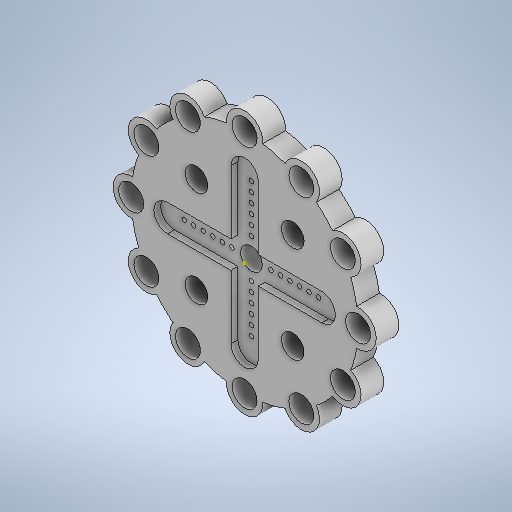
# Autodesk Inventor part: Servo_przelozenie
Saved by Autodesk Inventor 2025.2 (Build 292293000, 293)
## iProperties
Created: 2025-11-25
Part Number: Servo_przelozenie
Material: Ogólny
Document SubType Name: Modeling
Designer: juras
Density: 1 g/cm^3
Appearance: Domyślna
Author: juras
Autodesk Inventor part; units mm, degrees
ref_plane "YZ Plane" through (0, 0, 0) normal (1, 0, 0) x (0, 1, 0)
ref_plane "XZ Plane" through (0, 0, 0) normal (0, 1, 0) x (-1, 0, 0)
ref_plane "XY Plane" through (0, 0, 0) normal (0, 0, 1) x (1, 0, 0)
sketch "Szkic1" plane through (0, 0, 0) normal (0, 0, 1) x (1, 0, 0)
  circle A0 centre (0, 0) radius 25
  dimension "d0" = 50
  constraints: 1 centre point, 1 coincident
  measures "d0" diameter of A0
extrude "Wyciągnięcie proste1" add sketch "Szkic1" along normal mid plane 5
sketch "Szkic3" plane through (0, 0, 2.5) normal (0, 0, 1) x (1, 0, 0)
  point P0 (0, 0)
sketch "Szkic4" plane through (0, 0, 2.5) normal (0, 0, 1) x (1, 0, 0)
  circle A0 centre (0, 0) radius 2.4
  dimension "d3" = 4.8
  constraints: 1 centre point, 1 coincident
  measures "d3" diameter of A0
extrude "Wyciągnięcie proste2" cut sketch "Szkic4" against normal blind 5
sketch "Szkic7" plane through (0, 0, 2.5) normal (0, 0, 1) x (1, 0, 0)
  point P0 (0, 0)
sketch "Szkic11" plane through (0, 0, 2.5) normal (0, 0, 1) x (1, 0, 0)
  circle A0 centre (-25, 0) radius 4
  circle A1 centre (0, 0) radius 25 projected
  circle A2 centre (-21.6506, -12.5) radius 4
  circle A3 centre (-12.5, -21.6506) radius 4
  circle A4 centre (0, -25) radius 4
  circle A5 centre (12.5, -21.6506) radius 4
  circle A6 centre (21.6506, -12.5) radius 4
  circle A7 centre (25, 0) radius 4
  circle A8 centre (21.6506, 12.5) radius 4
  circle A9 centre (12.5, 21.6506) radius 4
  circle A10 centre (0, 25) radius 4
  circle A11 centre (-12.5, 21.6506) radius 4
  circle A12 centre (-21.6506, 12.5) radius 4
  point P0 (19.3799, 15.793)
  point P1 (23.3671, 8.887)
  point P2 (24.68, -3.9872)
  point P3 (24.68, 3.9872)
  point P4 (23.3671, -8.887)
  point P5 (19.3799, -15.793)
  point P6 (8.887, -23.3671)
  point P7 (15.793, -19.3799)
  point P8 (3.9872, -24.68)
  point P9 (-3.9872, -24.68)
  point P10 (-15.793, -19.3799)
  point P11 (-8.887, -23.3671)
  point P12 (-19.3799, -15.793)
  point P13 (-23.3671, -8.887)
  point P14 (-24.68, -3.9872)
  point P15 (-24.68, 3.9872)
  point P16 (8.887, 23.3671)
  point P17 (15.793, 19.3799)
  point P18 (-3.9872, 24.68)
  point P19 (3.9872, 24.68)
  point P20 (-15.793, 19.3799)
  point P21 (-8.887, 23.3671)
  point P22 (-23.3671, 8.887)
  point P23 (-19.3799, 15.793)
  dimension "d15" = 25
  dimension "d16" = 0
  dimension "d17" = 8
  dimension "d20" = 360
  constraints: 12 centre point, 26 other
  measures "d15" distance of point (0, 0) A0.centre
  measures "d16" vertical distance of point (0, 0) A0.centre
  measures "d17" diameter of A0
extrude "Wyciągnięcie proste3" add sketch "Szkic11" against normal blind 5
sketch "Szkic16" plane through (0, 0, 2.5) normal (0, 0, 1) x (1, 0, 0)
  arc A0 (-24.68, 3.9872) -> (-24.68, -3.9872) centre (-25, 0) ccw projected
  circle A1 centre (-25, 0) radius 2.75
  arc A2 (-24.68, 3.9872) -> (-24.68, -3.9872) centre (-25, 0) ccw projected
  point P0 (0, 0)
  dimension "d30" = 5.5
  constraints: 1 centre point, 1 coincident
  measures "d30" diameter of A1
extrude "Wyciągnięcie proste4" cut sketch "Szkic16" against normal blind 5.5
pattern_circular "Szyk kołowy1" count 12 over 360 about axis through (0, 0, 0) along (0, 0, 1) of "Wyciągnięcie proste4"
sketch "Szkic22" plane through (0, 0, 2.5) normal (0, 0, 1) x (1, 0, 0)
  line L0 (0, 0) -> (-4.3, 0)
  circle A0 centre (-4.3, 0) radius 0.5
  line L1 (-4.3, 0) -> (-6.4, 0)
  line L2 (-6.4, 0) -> (-8.5, 0)
  line L3 (-8.5, 0) -> (-10.6, 0)
  line L4 (-10.6, 0) -> (-12.7, 0)
  line L5 (-12.7, 0) -> (-14.8, 0)
  dimension "d51" = 4.3
  dimension "d52" = 1
  dimension "d53" = 2.1
  dimension "d54" = 2.1
  dimension "d55" = 2.1
  dimension "d56" = 2.1
  dimension "d57" = 2.1
  constraints: 12 end point, 5 point on line, 1 centre point, 1 coincident, 1 horizontal
  measures "d51" distance of L0.start L0.end
  measures "d52" diameter of A0
  measures "d53" distance of L1.start L1.end
  measures "d54" distance of L1.end L2.end
  measures "d55" distance of L2.end L3.end
  measures "d56" distance of L3.end L4.end
  measures "d57" distance of L4.end L5.end
hole "Otwór2" at (-14.8, 0, 2.5) at (-12.7, 0, 2.5) at (-10.6, 0, 2.5) at (-8.5, 0, 2.5) at (-6.4, 0, 2.5) at (-4.3, 0, 2.5) direction (0, 0, -1) diameter 1 depth 25 tip angle 118
pattern_circular "Szyk kołowy2" count 4 over 360 about axis through (0, 0, 0) along (0, 0, 1) of "Otwór2"
sketch "Szkic23" plane through (0, 0, 2.5) normal (0, 0, 1) x (1, 0, 0)
  circle A0 centre (0, 0) radius 3.75
  line L0 (0, 0) -> (3.75, 0) construction
  line L1 (-17, -3) -> (17, -3)
  line L2 (17, -3) -> (17, 3)
  line L3 (17, 3) -> (-17, 3)
  line L4 (-17, 3) -> (-17, -3)
  line L5 (-17, -3) -> (17, 3) construction
  line L6 (17, -3) -> (-17, 3) construction
  arc A1 (-17, 3) -> (-17, -3) centre (-17, 0) ccw
  arc A2 (17, -3) -> (17, 3) centre (17, 0) ccw
  point P0 (-2.25, -3)
  point P1 (2.25, -3)
  point P2 (2.25, 3)
  point P3 (-2.25, 3)
  dimension "d68" = 7.5
  dimension "d70" = 34
  dimension "d71" = 6
  constraints: 14 end point, 4 midpoint, 4 point on circle, 3 centre point, 2 horizontal, 2 parallel, 1 coincident, 1 perpendicular
  measures "d68" diameter of A0
  measures "d70" distance of L3.end L2.end
  measures "d71" distance of L2.end L1.end
extrude "Wyciągnięcie proste8" cut sketch "Szkic23" against normal blind 1.5
sketch "Szkic24" plane through (0, 0, 2.5) normal (0, 0, 1) x (1, 0, 0)
  line L0 (-3, -17) -> (3, -17)
  line L1 (3, -17) -> (3, 17)
  line L2 (3, 17) -> (-3, 17)
  line L3 (-3, 17) -> (-3, -17)
  line L4 (-3, -17) -> (3, 17) construction
  line L5 (3, -17) -> (-3, 17) construction
  arc A0 (2.8188, 15.9732) -> (-2.8188, 15.9732) centre (0, 17) ccw
  arc A1 (-2.8188, -15.9732) -> (2.8188, -15.9732) centre (0, -17) ccw
  point P0 (0, 0)
  point P1 (3, 17)
  point P2 (-3, 17)
  point P3 (-3, -17)
  point P4 (3, -17)
  point P5 (3, -17)
  point P6 (-3, -17)
  point P7 (-3, 17)
  point P8 (3, 17)
  dimension "d74" = 6
  dimension "d75" = 34
  dimension "d76" = 6
  dimension "d77" = 6
  constraints: 12 end point, 4 midpoint, 4 point on circle, 4 point on line, 2 centre point, 2 parallel, 1 horizontal, 1 perpendicular
  measures "d74" distance of L2.end L1.end
  measures "d75" distance of L1.end L0.end
  measures "d76" diameter of A0
  measures "d77" diameter of A1
extrude "Wyciągnięcie proste9" cut sketch "Szkic24" against normal blind 1.5
sketch "Szkic25" plane through (0, 0, 2.5) normal (0, 0, 1) x (1, 0, 0)
  line L0 (0, 0) -> (-10.6066, -10.6066)
  line L1 (0, 0) -> (15, 0) construction
  circle A0 centre (-10.6066, -10.6066) radius 2.5
  dimension "d80" = 15
  dimension "d81" = 135
  dimension "d82" = 5
  constraints: 4 end point, 1 centre point, 1 coincident, 1 equal length, 1 horizontal
  measures "d80" distance of L0.start L0.end
  measures "d81" angle of L0 L1
  measures "d82" diameter of A0
extrude "Wyciągnięcie proste10" cut sketch "Szkic25" against normal blind 5
pattern_circular "Szyk kołowy3" count 4 over 360 about axis through (0, 0, 0) along (0, 0, 1) of "Wyciągnięcie proste10"
sketch "Szkic26" plane through (0, 0, 1) normal (0, 0, 1) x (1, 0, 0)
  circle A0 centre (0, 0) radius 2.4
  dimension "d88" = 4.8
  constraints: 1 centre point, 1 coincident
  measures "d88" diameter of A0
extrude "Wyciągnięcie proste11" cut sketch "Szkic26" against normal blind 5
sketch "Szkic27" plane through (0, 0, 2.5) normal (0, 0, 1) x (1, 0, 0)
  point P0 (0, 0)
